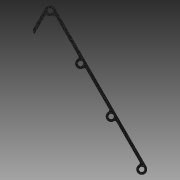
# Autodesk Inventor part: g16-strut2
Saved by Autodesk Inventor 2013 (Build 170138000, 138)
## iProperties
Created: 2013-03-23
Part Number: g16-strut2
Material: Acrylic
Document SubType Name: Modeling
Designer: Beth Scott
Density: 1 g/cm^3
Author: Beth Scott
Autodesk Inventor part; units mm, degrees
ref_plane "YZ Plane" through (0, 0, 0) normal (1, 0, 0) x (0, 1, 0)
ref_plane "XZ Plane" through (0, 0, 0) normal (0, 1, 0) x (-1, 0, 0)
ref_plane "XY Plane" through (0, 0, 0) normal (0, 0, 1) x (1, 0, 0)
sketch "LED Keepout Regions" plane through (0, 0, 0) normal (0, 0, 1) x (1, 0, 0)
  line L0 (115.0132, -121.5492) -> (110.0132, -121.5492) construction
  line L1 (110.0132, -121.5492) -> (110.0132, -116.5492) construction
  line L2 (110.0132, -116.5492) -> (115.0132, -116.5492) construction
  line L3 (115.0132, -116.5492) -> (115.0132, -121.5492) construction
  line L4 (112.5132, -124.1742) -> (112.5132, -113.9242) construction
  line L5 (120.8464, -119.0492) -> (104.1799, -119.0492) construction
  line L6 (109.5132, -122.0492) -> (107.0132, -122.0492) construction
  line L7 (107.0132, -122.0492) -> (107.0132, -116.0492) construction
  line L8 (107.0132, -116.0492) -> (109.5132, -116.0492) construction
  line L9 (109.5132, -116.0492) -> (109.5132, -122.0492) construction
  line L10 (120.8464, -124.1742) -> (104.1799, -124.1742) construction
  line L11 (104.1799, -124.1742) -> (104.1799, -113.9242) construction
  line L12 (104.1799, -113.9242) -> (120.8464, -113.9242) construction
  line L13 (120.8464, -113.9242) -> (120.8464, -124.1742) construction
  line L14 (117.0132, -113.9242) -> (117.0132, -124.1742) construction
  line L15 (105.0132, -113.9242) -> (105.0132, -124.1742) construction
  point P0 (111.5921, -119.1808)
  point P1 (115.0132, -119.0492)
  point P2 (112.5132, -121.5492)
  point P3 (109.5132, -119.0492)
  dimension "LED_StripWidth" = 10.25
  dimension "LED_Package" = 5
  dimension "LED_CapW" = 2.5
  dimension "LED_CapH" = 6
  dimension "d32" = 16.6665
  dimension "d52" = 2
  dimension "d53" = 2
  dimension "LED_CapDist" = 8
  measures "LED_StripWidth" distance of L12.end L10.start
  measures "LED_Package" distance of L0.start L0.end
  measures "LED_CapW" distance of L6.start L6.end
  measures "LED_CapH" distance of L6.end L7.end
  measures "d32" distance of L11.end L12.end
  measures "d52" distance between parallel lines of L7 L15
  measures "d53" distance between parallel lines of L14 L3
  measures "LED_CapDist" distance between parallel lines of L3 L7
sketch "LED Keepout x16" plane through (0, 0, 0) normal (0, 0, 1) x (1, 0, 0)
  line L0 (133.3347, -3) -> (0.0027, -3) construction
  line L1 (116.6682, -31.8672) -> (16.6692, -31.8672) construction
  line L2 (83.3352, -89.6017) -> (50.0022, -89.6017) construction
  line L3 (116.6682, -31.8672) -> (116.6682, -3) construction
  line L4 (100.0017, -60.7344) -> (33.3357, -60.7344) construction
  line L5 (100.0017, -60.7344) -> (100.0017, -31.8672) construction
  line L6 (83.3352, -89.6017) -> (83.3352, -60.7344) construction
  line L7 (66.6687, -118.4689) -> (66.6687, -89.6017) construction
  line L8 (50.0022, -89.6017) -> (50.0022, -3) construction
  line L9 (16.6692, -31.8672) -> (16.6692, -3) construction
  line L10 (33.3357, -60.7344) -> (33.3357, -3) construction
  line L11 (66.6687, -89.6017) -> (66.6687, -3) construction
  line L12 (83.3352, -60.7344) -> (83.3352, -3) construction
  line L13 (100.0017, -31.8672) -> (100.0017, -3) construction
  line L14 (102.5017, -19.9336) -> (97.5017, -19.9336) construction
  line L15 (97.5017, -19.9336) -> (97.5017, -14.9336) construction
  line L16 (97.5017, -14.9336) -> (102.5017, -14.9336) construction
  line L17 (102.5017, -14.9336) -> (102.5017, -19.9336) construction
  line L18 (100.0017, -22.5586) -> (100.0017, -12.3086) construction
  line L19 (108.335, -17.4336) -> (91.6685, -17.4336) construction
  line L20 (97.0017, -20.4336) -> (94.5017, -20.4336) construction
  line L21 (94.5017, -20.4336) -> (94.5017, -14.4336) construction
  line L22 (94.5017, -14.4336) -> (97.0017, -14.4336) construction
  line L23 (97.0017, -14.4336) -> (97.0017, -20.4336) construction
  line L24 (108.335, -22.5586) -> (91.6685, -22.5586) construction
  line L25 (91.6685, -22.5586) -> (91.6685, -12.3086) construction
  line L26 (91.6685, -12.3086) -> (108.335, -12.3086) construction
  line L27 (108.335, -12.3086) -> (108.335, -22.5586) construction
  line L28 (104.5017, -12.3086) -> (104.5017, -22.5586) construction
  line L29 (92.5017, -12.3086) -> (92.5017, -22.5586) construction
  line L30 (85.8352, -19.9336) -> (80.8352, -19.9336) construction
  line L31 (80.8352, -19.9336) -> (80.8352, -14.9336) construction
  line L32 (80.8352, -14.9336) -> (85.8352, -14.9336) construction
  line L33 (85.8352, -14.9336) -> (85.8352, -19.9336) construction
  line L34 (83.3352, -22.5586) -> (83.3352, -12.3086) construction
  line L35 (91.6685, -17.4336) -> (75.002, -17.4336) construction
  line L36 (80.3352, -20.4336) -> (77.8352, -20.4336) construction
  line L37 (77.8352, -20.4336) -> (77.8352, -14.4336) construction
  line L38 (77.8352, -14.4336) -> (80.3352, -14.4336) construction
  line L39 (80.3352, -14.4336) -> (80.3352, -20.4336) construction
  line L40 (91.6685, -22.5586) -> (75.002, -22.5586) construction
  line L41 (75.002, -22.5586) -> (75.002, -12.3086) construction
  line L42 (75.002, -12.3086) -> (91.6685, -12.3086) construction
  line L43 (91.6685, -12.3086) -> (91.6685, -22.5586) construction
  line L44 (87.8352, -12.3086) -> (87.8352, -22.5586) construction
  line L45 (75.8352, -12.3086) -> (75.8352, -22.5586) construction
  line L46 (69.1687, -19.9336) -> (64.1687, -19.9336) construction
  line L47 (64.1687, -19.9336) -> (64.1687, -14.9336) construction
  line L48 (64.1687, -14.9336) -> (69.1687, -14.9336) construction
  line L49 (69.1687, -14.9336) -> (69.1687, -19.9336) construction
  line L50 (66.6687, -22.5586) -> (66.6687, -12.3086) construction
  line L51 (75.002, -17.4336) -> (58.3355, -17.4336) construction
  line L52 (63.6687, -20.4336) -> (61.1687, -20.4336) construction
  line L53 (61.1687, -20.4336) -> (61.1687, -14.4336) construction
  line L54 (61.1687, -14.4336) -> (63.6687, -14.4336) construction
  line L55 (63.6687, -14.4336) -> (63.6687, -20.4336) construction
  line L56 (75.002, -22.5586) -> (58.3355, -22.5586) construction
  line L57 (58.3355, -22.5586) -> (58.3355, -12.3086) construction
  line L58 (58.3355, -12.3086) -> (75.002, -12.3086) construction
  line L59 (75.002, -12.3086) -> (75.002, -22.5586) construction
  line L60 (71.1687, -12.3086) -> (71.1687, -22.5586) construction
  line L61 (59.1687, -12.3086) -> (59.1687, -22.5586) construction
  line L62 (35.8357, -19.9336) -> (30.8357, -19.9336) construction
  line L63 (30.8357, -19.9336) -> (30.8357, -14.9336) construction
  line L64 (30.8357, -14.9336) -> (35.8357, -14.9336) construction
  line L65 (35.8357, -14.9336) -> (35.8357, -19.9336) construction
  line L66 (33.3357, -22.5586) -> (33.3357, -12.3086) construction
  line L67 (41.669, -17.4336) -> (25.0025, -17.4336) construction
  line L68 (30.3357, -20.4336) -> (27.8357, -20.4336) construction
  line L69 (27.8357, -20.4336) -> (27.8357, -14.4336) construction
  line L70 (27.8357, -14.4336) -> (30.3357, -14.4336) construction
  line L71 (30.3357, -14.4336) -> (30.3357, -20.4336) construction
  line L72 (41.669, -22.5586) -> (25.0025, -22.5586) construction
  line L73 (25.0025, -22.5586) -> (25.0025, -12.3086) construction
  line L74 (25.0025, -12.3086) -> (41.669, -12.3086) construction
  line L75 (41.669, -12.3086) -> (41.669, -22.5586) construction
  line L76 (37.8357, -12.3086) -> (37.8357, -22.5586) construction
  line L77 (25.8357, -12.3086) -> (25.8357, -22.5586) construction
  line L78 (52.5022, -19.9336) -> (47.5022, -19.9336) construction
  line L79 (47.5022, -19.9336) -> (47.5022, -14.9336) construction
  line L80 (47.5022, -14.9336) -> (52.5022, -14.9336) construction
  line L81 (52.5022, -14.9336) -> (52.5022, -19.9336) construction
  line L82 (50.0022, -22.5586) -> (50.0022, -12.3086) construction
  line L83 (58.3355, -17.4336) -> (41.669, -17.4336) construction
  line L84 (47.0022, -20.4336) -> (44.5022, -20.4336) construction
  line L85 (44.5022, -20.4336) -> (44.5022, -14.4336) construction
  line L86 (44.5022, -14.4336) -> (47.0022, -14.4336) construction
  line L87 (47.0022, -14.4336) -> (47.0022, -20.4336) construction
  line L88 (58.3355, -22.5586) -> (41.669, -22.5586) construction
  line L89 (41.669, -22.5586) -> (41.669, -12.3086) construction
  line L90 (41.669, -12.3086) -> (58.3355, -12.3086) construction
  line L91 (58.3355, -12.3086) -> (58.3355, -22.5586) construction
  line L92 (54.5022, -12.3086) -> (54.5022, -22.5586) construction
  line L93 (42.5022, -12.3086) -> (42.5022, -22.5586) construction
  line L94 (19.1692, -19.9336) -> (14.1692, -19.9336) construction
  line L95 (14.1692, -19.9336) -> (14.1692, -14.9336) construction
  line L96 (14.1692, -14.9336) -> (19.1692, -14.9336) construction
  line L97 (19.1692, -14.9336) -> (19.1692, -19.9336) construction
  line L98 (16.6692, -22.5586) -> (16.6692, -12.3086) construction
  line L99 (25.0025, -17.4336) -> (8.336, -17.4336) construction
  line L100 (13.6692, -20.4336) -> (11.1692, -20.4336) construction
  line L101 (11.1692, -20.4336) -> (11.1692, -14.4336) construction
  line L102 (11.1692, -14.4336) -> (13.6692, -14.4336) construction
  line L103 (13.6692, -14.4336) -> (13.6692, -20.4336) construction
  line L104 (25.0025, -22.5586) -> (8.336, -22.5586) construction
  line L105 (8.336, -22.5586) -> (8.336, -12.3086) construction
  line L106 (8.336, -12.3086) -> (25.0025, -12.3086) construction
  line L107 (25.0025, -12.3086) -> (25.0025, -22.5586) construction
  line L108 (21.1692, -12.3086) -> (21.1692, -22.5586) construction
  line L109 (9.1692, -12.3086) -> (9.1692, -22.5586) construction
  line L110 (69.1687, -77.6681) -> (64.1687, -77.6681) construction
  line L111 (64.1687, -77.6681) -> (64.1687, -72.6681) construction
  line L112 (64.1687, -72.6681) -> (69.1687, -72.6681) construction
  line L113 (69.1687, -72.6681) -> (69.1687, -77.6681) construction
  line L114 (66.6687, -80.2931) -> (66.6687, -70.0431) construction
  line L115 (75.002, -75.1681) -> (58.3355, -75.1681) construction
  line L116 (63.6687, -78.1681) -> (61.1687, -78.1681) construction
  line L117 (61.1687, -78.1681) -> (61.1687, -72.1681) construction
  line L118 (61.1687, -72.1681) -> (63.6687, -72.1681) construction
  line L119 (63.6687, -72.1681) -> (63.6687, -78.1681) construction
  line L120 (75.002, -80.2931) -> (58.3355, -80.2931) construction
  line L121 (58.3355, -80.2931) -> (58.3355, -70.0431) construction
  line L122 (58.3355, -70.0431) -> (75.002, -70.0431) construction
  line L123 (75.002, -70.0431) -> (75.002, -80.2931) construction
  line L124 (71.1687, -70.0431) -> (71.1687, -80.2931) construction
  line L125 (59.1687, -70.0431) -> (59.1687, -80.2931) construction
  line L126 (52.5022, -77.6681) -> (47.5022, -77.6681) construction
  line L127 (47.5022, -77.6681) -> (47.5022, -72.6681) construction
  line L128 (47.5022, -72.6681) -> (52.5022, -72.6681) construction
  line L129 (52.5022, -72.6681) -> (52.5022, -77.6681) construction
  line L130 (50.0022, -80.2931) -> (50.0022, -70.0431) construction
  line L131 (58.3355, -75.1681) -> (41.669, -75.1681) construction
  line L132 (47.0022, -78.1681) -> (44.5022, -78.1681) construction
  line L133 (44.5022, -78.1681) -> (44.5022, -72.1681) construction
  line L134 (44.5022, -72.1681) -> (47.0022, -72.1681) construction
  line L135 (47.0022, -72.1681) -> (47.0022, -78.1681) construction
  line L136 (58.3355, -80.2931) -> (41.669, -80.2931) construction
  line L137 (41.669, -80.2931) -> (41.669, -70.0431) construction
  line L138 (41.669, -70.0431) -> (58.3355, -70.0431) construction
  line L139 (58.3355, -70.0431) -> (58.3355, -80.2931) construction
  line L140 (54.5022, -70.0431) -> (54.5022, -80.2931) construction
  line L141 (42.5022, -70.0431) -> (42.5022, -80.2931) construction
  line L142 (30.8357, -43.8008) -> (35.8357, -43.8008) construction
  line L143 (35.8357, -43.8008) -> (35.8357, -48.8008) construction
  line L144 (35.8357, -48.8008) -> (30.8357, -48.8008) construction
  line L145 (30.8357, -48.8008) -> (30.8357, -43.8008) construction
  line L146 (33.3357, -41.1758) -> (33.3357, -51.4258) construction
  line L147 (25.0025, -46.3008) -> (41.669, -46.3008) construction
  line L148 (36.3357, -43.3008) -> (38.8357, -43.3008) construction
  line L149 (38.8357, -43.3008) -> (38.8357, -49.3008) construction
  line L150 (38.8357, -49.3008) -> (36.3357, -49.3008) construction
  line L151 (36.3357, -49.3008) -> (36.3357, -43.3008) construction
  line L152 (25.0025, -41.1758) -> (41.669, -41.1758) construction
  line L153 (41.669, -41.1758) -> (41.669, -51.4258) construction
  line L154 (41.669, -51.4258) -> (25.0025, -51.4258) construction
  line L155 (25.0025, -51.4258) -> (25.0025, -41.1758) construction
  line L156 (28.8357, -51.4258) -> (28.8357, -41.1758) construction
  line L157 (40.8357, -51.4258) -> (40.8357, -41.1758) construction
  line L158 (85.8352, -77.6681) -> (80.8352, -77.6681) construction
  line L159 (80.8352, -77.6681) -> (80.8352, -72.6681) construction
  line L160 (80.8352, -72.6681) -> (85.8352, -72.6681) construction
  line L161 (85.8352, -72.6681) -> (85.8352, -77.6681) construction
  line L162 (83.3352, -80.2931) -> (83.3352, -70.0431) construction
  line L163 (91.6685, -75.1681) -> (75.002, -75.1681) construction
  line L164 (80.3352, -78.1681) -> (77.8352, -78.1681) construction
  line L165 (77.8352, -78.1681) -> (77.8352, -72.1681) construction
  line L166 (77.8352, -72.1681) -> (80.3352, -72.1681) construction
  line L167 (80.3352, -72.1681) -> (80.3352, -78.1681) construction
  line L168 (91.6685, -80.2931) -> (75.002, -80.2931) construction
  line L169 (75.002, -80.2931) -> (75.002, -70.0431) construction
  line L170 (75.002, -70.0431) -> (91.6685, -70.0431) construction
  line L171 (91.6685, -70.0431) -> (91.6685, -80.2931) construction
  line L172 (87.8352, -70.0431) -> (87.8352, -80.2931) construction
  line L173 (75.8352, -70.0431) -> (75.8352, -80.2931) construction
  line L174 (64.1687, -43.8008) -> (69.1687, -43.8008) construction
  line L175 (69.1687, -43.8008) -> (69.1687, -48.8008) construction
  line L176 (69.1687, -48.8008) -> (64.1687, -48.8008) construction
  line L177 (64.1687, -48.8008) -> (64.1687, -43.8008) construction
  line L178 (66.6687, -41.1758) -> (66.6687, -51.4258) construction
  line L179 (58.3355, -46.3008) -> (75.002, -46.3008) construction
  line L180 (69.6687, -43.3008) -> (72.1687, -43.3008) construction
  line L181 (72.1687, -43.3008) -> (72.1687, -49.3008) construction
  line L182 (72.1687, -49.3008) -> (69.6687, -49.3008) construction
  line L183 (69.6687, -49.3008) -> (69.6687, -43.3008) construction
  line L184 (58.3355, -41.1758) -> (75.002, -41.1758) construction
  line L185 (75.002, -41.1758) -> (75.002, -51.4258) construction
  line L186 (75.002, -51.4258) -> (58.3355, -51.4258) construction
  line L187 (58.3355, -51.4258) -> (58.3355, -41.1758) construction
  line L188 (62.1687, -51.4258) -> (62.1687, -41.1758) construction
  line L189 (74.1687, -51.4258) -> (74.1687, -41.1758) construction
  line L190 (80.8352, -43.8008) -> (85.8352, -43.8008) construction
  line L191 (85.8352, -43.8008) -> (85.8352, -48.8008) construction
  line L192 (85.8352, -48.8008) -> (80.8352, -48.8008) construction
  line L193 (80.8352, -48.8008) -> (80.8352, -43.8008) construction
  line L194 (83.3352, -41.1758) -> (83.3352, -51.4258) construction
  line L195 (75.002, -46.3008) -> (91.6685, -46.3008) construction
  line L196 (86.3352, -43.3008) -> (88.8352, -43.3008) construction
  line L197 (88.8352, -43.3008) -> (88.8352, -49.3008) construction
  line L198 (88.8352, -49.3008) -> (86.3352, -49.3008) construction
  line L199 (86.3352, -49.3008) -> (86.3352, -43.3008) construction
  line L200 (75.002, -41.1758) -> (91.6685, -41.1758) construction
  line L201 (91.6685, -41.1758) -> (91.6685, -51.4258) construction
  line L202 (91.6685, -51.4258) -> (75.002, -51.4258) construction
  line L203 (75.002, -51.4258) -> (75.002, -41.1758) construction
  line L204 (78.8352, -51.4258) -> (78.8352, -41.1758) construction
  line L205 (90.8352, -51.4258) -> (90.8352, -41.1758) construction
  line L206 (47.5022, -43.8008) -> (52.5022, -43.8008) construction
  line L207 (52.5022, -43.8008) -> (52.5022, -48.8008) construction
  line L208 (52.5022, -48.8008) -> (47.5022, -48.8008) construction
  line L209 (47.5022, -48.8008) -> (47.5022, -43.8008) construction
  line L210 (50.0022, -41.1758) -> (50.0022, -51.4258) construction
  line L211 (41.669, -46.3008) -> (58.3355, -46.3008) construction
  line L212 (53.0022, -43.3008) -> (55.5022, -43.3008) construction
  line L213 (55.5022, -43.3008) -> (55.5022, -49.3008) construction
  line L214 (55.5022, -49.3008) -> (53.0022, -49.3008) construction
  line L215 (53.0022, -49.3008) -> (53.0022, -43.3008) construction
  line L216 (41.669, -41.1758) -> (58.3355, -41.1758) construction
  line L217 (58.3355, -41.1758) -> (58.3355, -51.4258) construction
  line L218 (58.3355, -51.4258) -> (41.669, -51.4258) construction
  line L219 (41.669, -51.4258) -> (41.669, -41.1758) construction
  line L220 (45.5022, -51.4258) -> (45.5022, -41.1758) construction
  line L221 (57.5022, -51.4258) -> (57.5022, -41.1758) construction
  line L222 (97.5017, -43.8008) -> (102.5017, -43.8008) construction
  line L223 (102.5017, -43.8008) -> (102.5017, -48.8008) construction
  line L224 (102.5017, -48.8008) -> (97.5017, -48.8008) construction
  line L225 (97.5017, -48.8008) -> (97.5017, -43.8008) construction
  line L226 (100.0017, -41.1758) -> (100.0017, -51.4258) construction
  line L227 (91.6685, -46.3008) -> (108.335, -46.3008) construction
  line L228 (103.0017, -43.3008) -> (105.5017, -43.3008) construction
  line L229 (105.5017, -43.3008) -> (105.5017, -49.3008) construction
  line L230 (105.5017, -49.3008) -> (103.0017, -49.3008) construction
  line L231 (103.0017, -49.3008) -> (103.0017, -43.3008) construction
  line L232 (91.6685, -41.1758) -> (108.335, -41.1758) construction
  line L233 (108.335, -41.1758) -> (108.335, -51.4258) construction
  line L234 (108.335, -51.4258) -> (91.6685, -51.4258) construction
  line L235 (91.6685, -51.4258) -> (91.6685, -41.1758) construction
  line L236 (95.5017, -51.4258) -> (95.5017, -41.1758) construction
  line L237 (107.5017, -51.4258) -> (107.5017, -41.1758) construction
  line L238 (64.1687, -101.5353) -> (69.1687, -101.5353) construction
  line L239 (69.1687, -101.5353) -> (69.1687, -106.5353) construction
  line L240 (69.1687, -106.5353) -> (64.1687, -106.5353) construction
  line L241 (64.1687, -106.5353) -> (64.1687, -101.5353) construction
  line L242 (66.6687, -98.9103) -> (66.6687, -109.1603) construction
  line L243 (58.3355, -104.0353) -> (75.002, -104.0353) construction
  line L244 (69.6687, -101.0353) -> (72.1687, -101.0353) construction
  line L245 (72.1687, -101.0353) -> (72.1687, -107.0353) construction
  line L246 (72.1687, -107.0353) -> (69.6687, -107.0353) construction
  line L247 (69.6687, -107.0353) -> (69.6687, -101.0353) construction
  line L248 (58.3355, -98.9103) -> (75.002, -98.9103) construction
  line L249 (75.002, -98.9103) -> (75.002, -109.1603) construction
  line L250 (75.002, -109.1603) -> (58.3355, -109.1603) construction
  line L251 (58.3355, -109.1603) -> (58.3355, -98.9103) construction
  line L252 (62.1687, -109.1603) -> (62.1687, -98.9103) construction
  line L253 (74.1687, -109.1603) -> (74.1687, -98.9103) construction
  line L254 (119.1682, -19.9336) -> (114.1682, -19.9336) construction
  line L255 (114.1682, -19.9336) -> (114.1682, -14.9336) construction
  line L256 (114.1682, -14.9336) -> (119.1682, -14.9336) construction
  line L257 (119.1682, -14.9336) -> (119.1682, -19.9336) construction
  line L258 (116.6682, -22.5586) -> (116.6682, -12.3086) construction
  line L259 (125.0015, -17.4336) -> (108.335, -17.4336) construction
  line L260 (113.6682, -20.4336) -> (111.1682, -20.4336) construction
  line L261 (111.1682, -20.4336) -> (111.1682, -14.4336) construction
  line L262 (111.1682, -14.4336) -> (113.6682, -14.4336) construction
  line L263 (113.6682, -14.4336) -> (113.6682, -20.4336) construction
  line L264 (125.0015, -22.5586) -> (108.335, -22.5586) construction
  line L265 (108.335, -22.5586) -> (108.335, -12.3086) construction
  line L266 (108.335, -12.3086) -> (125.0015, -12.3086) construction
  line L267 (125.0015, -12.3086) -> (125.0015, -22.5586) construction
  line L268 (121.1682, -12.3086) -> (121.1682, -22.5586) construction
  line L269 (109.1682, -12.3086) -> (109.1682, -22.5586) construction
  point P0 (73.3279, -41.0278)
  point P1 (116.6682, -17.4336)
  point P2 (116.6682, -17.4336)
  point P3 (100.0017, -17.4336)
  point P4 (100.0017, -17.4336)
  point P5 (83.3352, -75.1681)
  point P6 (100.0017, -46.3008)
  point P7 (66.6687, -104.0353)
  point P8 (83.3352, -17.4336)
  point P9 (66.6687, -17.4336)
  point P10 (33.3357, -17.4336)
  point P11 (16.6692, -17.4336)
  point P12 (100.0017, -46.3008)
  point P13 (83.3352, -46.3008)
  point P14 (66.6687, -46.3008)
  point P15 (50.0022, -46.3008)
  point P16 (33.3357, -46.3008)
  point P17 (50.0022, -75.1681)
  point P18 (66.6687, -75.1681)
  point P19 (83.3352, -75.1681)
  point P20 (66.6687, -104.0353)
  dimension "d56" = 16.6665
  dimension "d61" = 16.6665
  dimension "d62" = 28.8672
  measures "d56" distance from line of L9 L0.end
  measures "d61" distance from line of L0.start L3
  measures "d62" distance of L1.end L9.end
derived "g16-strut1.ipt"
sketch "Strut Templates" plane through (0, 0, 0) normal (0, 1, 0) x (-1, 0, 0)
  circle A0 centre (16.6665, 28.8672) radius 1.5
  circle A1 centre (33.333, 57.7344) radius 1.5
  circle A2 centre (0, 0) radius 1.5
  circle A3 centre (33.333, 0) radius 1.5
  circle A4 centre (66.666, 0) radius 1.5
  circle A5 centre (99.999, 0) radius 1.5
  circle A6 centre (133.332, 0) radius 1.5
  circle A7 centre (116.6655, 28.8672) radius 1.5
  circle A8 centre (99.999, 57.7344) radius 1.5
  circle A9 centre (83.3325, 86.6017) radius 1.5
  circle A10 centre (49.9995, 86.6017) radius 1.5
  circle A11 centre (66.666, 115.4689) radius 1.5
  arc A12 (-2.5981, 1.5) -> (0, -3) centre (0, 0) ccw
  line L0 (0, -3) -> (133.332, -3)
  arc A13 (36.333, 0) -> (30.333, 0) centre (33.333, 0) ccw
  arc A14 (69.666, 0) -> (66.666, -3) centre (66.666, 0) ccw
  circle A15 centre (49.9995, 86.6017) radius 3 construction
  line L1 (-2.5981, 1.5) -> (57.2344, 105.1329)
  circle A16 centre (16.6665, 28.8672) radius 3 construction
  circle A17 centre (33.333, 57.7344) radius 3 construction
  line L2 (29.333, -1) -> (4, -1)
  arc A18 (29.333, -1) -> (30.333, 0) centre (29.333, 0) ccw
  circle A19 centre (0, 0) radius 3 construction
  arc A20 (3, 0) -> (1.5, 2.5981) centre (0, 0) ccw
  arc A21 (3, 0) -> (4, -1) centre (4, 0) ccw
  arc A22 (1.134, 3.9641) -> (1.5, 2.5981) centre (2, 3.4641) ccw
  line L3 (1.134, 3.9641) -> (13.8005, 25.9031)
  arc A23 (15.1665, 26.2691) -> (13.8005, 25.9031) centre (14.6665, 25.4031) ccw
  arc A24 (15.1665, 26.2691) -> (18.1665, 31.4653) centre (16.6665, 28.8672) ccw
  arc A25 (17.8005, 32.8313) -> (18.1665, 31.4653) centre (18.6665, 32.3313) ccw
  line L4 (17.8005, 32.8313) -> (30.467, 54.7703)
  line L5 (34.467, 61.6986) -> (47.1335, 83.6376)
  arc A26 (31.833, 55.1364) -> (34.833, 60.3325) centre (33.333, 57.7344) ccw
  arc A27 (34.467, 61.6986) -> (34.833, 60.3325) centre (35.333, 61.1986) ccw
  arc A28 (31.833, 55.1364) -> (30.467, 54.7703) centre (31.333, 54.2703) ccw
  arc A29 (51.1335, 90.5658) -> (51.4995, 89.1998) centre (51.9995, 90.0658) ccw
  arc A30 (48.4995, 84.0036) -> (51.4995, 89.1998) centre (49.9995, 86.6017) ccw
  arc A31 (48.4995, 84.0036) -> (47.1335, 83.6376) centre (47.9995, 83.1376) ccw
  arc A32 (69.2641, 116.9689) -> (64.0679, 116.9689) centre (66.666, 115.4689) ccw
  line L6 (64.0679, 116.9689) -> (57.235, 105.1339)
  line L7 (51.1335, 90.5658) -> (57.9664, 102.4008)
  line L8 (57.235, 105.1339) -> (57.967, 102.4018)
  line L9 (57.967, 102.4018) -> (63.8, 112.5048)
  line L10 (57.9664, 102.4008) -> (57.2344, 105.1329)
  arc A33 (65.166, 112.8708) -> (68.166, 112.8708) centre (66.666, 115.4689) ccw
  arc A34 (65.166, 112.8708) -> (63.8, 112.5048) centre (64.666, 112.0048) ccw
  arc A35 (133.332, -3) -> (130.332, 0) centre (133.332, 0) ccw
  line L11 (66.666, -3) -> (133.332, -3)
  line L12 (69.2641, 116.9689) -> (119.2636, 30.3672)
  arc A36 (102.999, 0) -> (96.999, 0) centre (99.999, 0) ccw
  arc A37 (131.832, 2.5981) -> (130.332, 0) centre (133.332, 0) ccw
  arc A38 (115.1655, 31.4653) -> (119.2636, 30.3672) centre (116.6655, 28.8672) ccw
  arc A39 (98.499, 60.3325) -> (101.499, 55.1364) centre (99.999, 57.7344) ccw
  arc A40 (81.8325, 89.1998) -> (84.8325, 84.0036) centre (83.3325, 86.6017) ccw
  line L13 (70.666, -1) -> (95.999, -1)
  line L14 (103.999, -1) -> (129.332, -1)
  line L15 (132.198, 3.9641) -> (119.5315, 25.9031)
  line L16 (115.5315, 32.8313) -> (102.865, 54.7703)
  line L17 (98.865, 61.6986) -> (86.1985, 83.6376)
  line L18 (82.1985, 90.5658) -> (69.532, 112.5048)
  arc A41 (69.666, 0) -> (70.666, -1) centre (70.666, 0) ccw
  arc A42 (95.999, -1) -> (96.999, 0) centre (95.999, 0) ccw
  arc A43 (102.999, 0) -> (103.999, -1) centre (103.999, 0) ccw
  arc A44 (129.332, -1) -> (130.332, 0) centre (129.332, 0) ccw
  arc A45 (69.532, 112.5048) -> (68.166, 112.8708) centre (68.666, 112.0048) ccw
  arc A46 (81.8325, 89.1998) -> (82.1985, 90.5658) centre (81.3325, 90.0658) ccw
  arc A47 (86.1985, 83.6376) -> (84.8325, 84.0036) centre (85.3325, 83.1376) ccw
  arc A48 (98.499, 60.3325) -> (98.865, 61.6986) centre (97.999, 61.1986) ccw
  arc A49 (102.865, 54.7703) -> (101.499, 55.1364) centre (101.999, 54.2703) ccw
  arc A50 (119.5315, 25.9031) -> (118.1655, 26.2691) centre (118.6655, 25.4031) ccw
  arc A51 (115.1655, 31.4653) -> (115.5315, 32.8313) centre (114.6655, 32.3313) ccw
  arc A52 (131.832, 2.5981) -> (132.198, 3.9641) centre (131.332, 3.4641) ccw
  line L19 (37.333, -1) -> (62.666, -1)
  arc A53 (36.333, 0) -> (37.333, -1) centre (37.333, 0) ccw
  arc A54 (62.666, -1) -> (63.666, 0) centre (62.666, 0) ccw
  arc A55 (69.666, 0) -> (63.666, 0) centre (66.666, 0) ccw
  line L20 (0, 0) -> (133.332, 0) construction
  line L21 (16.6665, 28.8672) -> (116.6655, 28.8672) construction
  line L22 (49.9995, 86.6017) -> (83.3325, 86.6017) construction
  line L23 (16.6665, 28.8672) -> (16.6665, 0) construction
  line L24 (33.333, 57.7344) -> (99.999, 57.7344) construction
  line L25 (33.333, 57.7344) -> (33.333, 28.8672) construction
  line L26 (49.9995, 86.6017) -> (49.9995, 57.7344) construction
  line L27 (66.666, 115.4689) -> (66.666, 86.6017) construction
  line L28 (83.3325, 86.6017) -> (83.3325, 0) construction
  line L29 (116.6655, 28.8672) -> (116.6655, 0) construction
  line L30 (99.999, 57.7344) -> (99.999, 0) construction
  line L31 (66.666, 86.6017) -> (66.666, 0) construction
  line L32 (49.9995, 57.7344) -> (49.9995, 0) construction
  line L33 (33.333, 28.8672) -> (33.333, 0) construction
  line L34 (30.833, 16.9336) -> (35.833, 16.9336) construction
  line L35 (35.833, 16.9336) -> (35.833, 11.9336) construction
  line L36 (35.833, 11.9336) -> (30.833, 11.9336) construction
  line L37 (30.833, 11.9336) -> (30.833, 16.9336) construction
  line L38 (33.333, 19.5586) -> (33.333, 9.3086) construction
  line L39 (24.9998, 14.4336) -> (41.6663, 14.4336) construction
  line L40 (36.333, 17.4336) -> (38.833, 17.4336) construction
  line L41 (38.833, 17.4336) -> (38.833, 11.4336) construction
  line L42 (38.833, 11.4336) -> (36.333, 11.4336) construction
  line L43 (36.333, 11.4336) -> (36.333, 17.4336) construction
  line L44 (24.9998, 19.5586) -> (41.6663, 19.5586) construction
  line L45 (41.6663, 19.5586) -> (41.6663, 9.3086) construction
  line L46 (41.6663, 9.3086) -> (24.9998, 9.3086) construction
  line L47 (24.9998, 9.3086) -> (24.9998, 19.5586) construction
  line L48 (28.833, 9.3086) -> (28.833, 19.5586) construction
  line L49 (40.833, 9.3086) -> (40.833, 19.5586) construction
  line L50 (47.4995, 16.9336) -> (52.4995, 16.9336) construction
  line L51 (52.4995, 16.9336) -> (52.4995, 11.9336) construction
  line L52 (52.4995, 11.9336) -> (47.4995, 11.9336) construction
  line L53 (47.4995, 11.9336) -> (47.4995, 16.9336) construction
  line L54 (49.9995, 19.5586) -> (49.9995, 9.3086) construction
  line L55 (41.6663, 14.4336) -> (58.3328, 14.4336) construction
  line L56 (52.9995, 17.4336) -> (55.4995, 17.4336) construction
  line L57 (55.4995, 17.4336) -> (55.4995, 11.4336) construction
  line L58 (55.4995, 11.4336) -> (52.9995, 11.4336) construction
  line L59 (52.9995, 11.4336) -> (52.9995, 17.4336) construction
  line L60 (41.6663, 19.5586) -> (58.3328, 19.5586) construction
  line L61 (58.3328, 19.5586) -> (58.3328, 9.3086) construction
  line L62 (58.3328, 9.3086) -> (41.6663, 9.3086) construction
  line L63 (41.6663, 9.3086) -> (41.6663, 19.5586) construction
  line L64 (45.4995, 9.3086) -> (45.4995, 19.5586) construction
  line L65 (57.4995, 9.3086) -> (57.4995, 19.5586) construction
  line L66 (64.166, 16.9336) -> (69.166, 16.9336) construction
  line L67 (69.166, 16.9336) -> (69.166, 11.9336) construction
  line L68 (69.166, 11.9336) -> (64.166, 11.9336) construction
  line L69 (64.166, 11.9336) -> (64.166, 16.9336) construction
  line L70 (66.666, 19.5586) -> (66.666, 9.3086) construction
  line L71 (58.3328, 14.4336) -> (74.9993, 14.4336) construction
  line L72 (69.666, 17.4336) -> (72.166, 17.4336) construction
  line L73 (72.166, 17.4336) -> (72.166, 11.4336) construction
  line L74 (72.166, 11.4336) -> (69.666, 11.4336) construction
  line L75 (69.666, 11.4336) -> (69.666, 17.4336) construction
  line L76 (58.3328, 19.5586) -> (74.9993, 19.5586) construction
  line L77 (74.9993, 19.5586) -> (74.9993, 9.3086) construction
  line L78 (74.9993, 9.3086) -> (58.3328, 9.3086) construction
  line L79 (58.3328, 9.3086) -> (58.3328, 19.5586) construction
  line L80 (62.166, 9.3086) -> (62.166, 19.5586) construction
  line L81 (74.166, 9.3086) -> (74.166, 19.5586) construction
  line L82 (97.499, 16.9336) -> (102.499, 16.9336) construction
  line L83 (102.499, 16.9336) -> (102.499, 11.9336) construction
  line L84 (102.499, 11.9336) -> (97.499, 11.9336) construction
  line L85 (97.499, 11.9336) -> (97.499, 16.9336) construction
  line L86 (99.999, 19.5586) -> (99.999, 9.3086) construction
  line L87 (91.6658, 14.4336) -> (108.3323, 14.4336) construction
  line L88 (102.999, 17.4336) -> (105.499, 17.4336) construction
  line L89 (105.499, 17.4336) -> (105.499, 11.4336) construction
  line L90 (105.499, 11.4336) -> (102.999, 11.4336) construction
  line L91 (102.999, 11.4336) -> (102.999, 17.4336) construction
  line L92 (91.6658, 19.5586) -> (108.3323, 19.5586) construction
  line L93 (108.3323, 19.5586) -> (108.3323, 9.3086) construction
  line L94 (108.3323, 9.3086) -> (91.6658, 9.3086) construction
  line L95 (91.6658, 9.3086) -> (91.6658, 19.5586) construction
  line L96 (95.499, 9.3086) -> (95.499, 19.5586) construction
  line L97 (107.499, 9.3086) -> (107.499, 19.5586) construction
  line L98 (80.8325, 16.9336) -> (85.8325, 16.9336) construction
  line L99 (85.8325, 16.9336) -> (85.8325, 11.9336) construction
  line L100 (85.8325, 11.9336) -> (80.8325, 11.9336) construction
  line L101 (80.8325, 11.9336) -> (80.8325, 16.9336) construction
  line L102 (83.3325, 19.5586) -> (83.3325, 9.3086) construction
  line L103 (74.9993, 14.4336) -> (91.6658, 14.4336) construction
  line L104 (86.3325, 17.4336) -> (88.8325, 17.4336) construction
  line L105 (88.8325, 17.4336) -> (88.8325, 11.4336) construction
  line L106 (88.8325, 11.4336) -> (86.3325, 11.4336) construction
  line L107 (86.3325, 11.4336) -> (86.3325, 17.4336) construction
  line L108 (74.9993, 19.5586) -> (91.6658, 19.5586) construction
  line L109 (91.6658, 19.5586) -> (91.6658, 9.3086) construction
  line L110 (91.6658, 9.3086) -> (74.9993, 9.3086) construction
  line L111 (74.9993, 9.3086) -> (74.9993, 19.5586) construction
  line L112 (78.8325, 9.3086) -> (78.8325, 19.5586) construction
  line L113 (90.8325, 9.3086) -> (90.8325, 19.5586) construction
  line L114 (114.1655, 16.9336) -> (119.1655, 16.9336) construction
  line L115 (119.1655, 16.9336) -> (119.1655, 11.9336) construction
  line L116 (119.1655, 11.9336) -> (114.1655, 11.9336) construction
  line L117 (114.1655, 11.9336) -> (114.1655, 16.9336) construction
  line L118 (116.6655, 19.5586) -> (116.6655, 9.3086) construction
  line L119 (108.3323, 14.4336) -> (124.9988, 14.4336) construction
  line L120 (119.6655, 17.4336) -> (122.1655, 17.4336) construction
  line L121 (122.1655, 17.4336) -> (122.1655, 11.4336) construction
  line L122 (122.1655, 11.4336) -> (119.6655, 11.4336) construction
  line L123 (119.6655, 11.4336) -> (119.6655, 17.4336) construction
  line L124 (108.3323, 19.5586) -> (124.9988, 19.5586) construction
  line L125 (124.9988, 19.5586) -> (124.9988, 9.3086) construction
  line L126 (124.9988, 9.3086) -> (108.3323, 9.3086) construction
  line L127 (108.3323, 9.3086) -> (108.3323, 19.5586) construction
  line L128 (112.1655, 9.3086) -> (112.1655, 19.5586) construction
  line L129 (124.1655, 9.3086) -> (124.1655, 19.5586) construction
  line L130 (64.166, 74.6681) -> (69.166, 74.6681) construction
  line L131 (69.166, 74.6681) -> (69.166, 69.6681) construction
  line L132 (69.166, 69.6681) -> (64.166, 69.6681) construction
  line L133 (64.166, 69.6681) -> (64.166, 74.6681) construction
  line L134 (66.666, 77.2931) -> (66.666, 67.0431) construction
  line L135 (58.3328, 72.1681) -> (74.9993, 72.1681) construction
  line L136 (69.666, 75.1681) -> (72.166, 75.1681) construction
  line L137 (72.166, 75.1681) -> (72.166, 69.1681) construction
  line L138 (72.166, 69.1681) -> (69.666, 69.1681) construction
  line L139 (69.666, 69.1681) -> (69.666, 75.1681) construction
  line L140 (58.3328, 77.2931) -> (74.9993, 77.2931) construction
  line L141 (74.9993, 77.2931) -> (74.9993, 67.0431) construction
  line L142 (74.9993, 67.0431) -> (58.3328, 67.0431) construction
  line L143 (58.3328, 67.0431) -> (58.3328, 77.2931) construction
  line L144 (62.166, 67.0431) -> (62.166, 77.2931) construction
  line L145 (74.166, 67.0431) -> (74.166, 77.2931) construction
  line L146 (80.8325, 74.6681) -> (85.8325, 74.6681) construction
  line L147 (85.8325, 74.6681) -> (85.8325, 69.6681) construction
  line L148 (85.8325, 69.6681) -> (80.8325, 69.6681) construction
  line L149 (80.8325, 69.6681) -> (80.8325, 74.6681) construction
  line L150 (83.3325, 77.2931) -> (83.3325, 67.0431) construction
  line L151 (74.9993, 72.1681) -> (91.6658, 72.1681) construction
  line L152 (86.3325, 75.1681) -> (88.8325, 75.1681) construction
  line L153 (88.8325, 75.1681) -> (88.8325, 69.1681) construction
  line L154 (88.8325, 69.1681) -> (86.3325, 69.1681) construction
  line L155 (86.3325, 69.1681) -> (86.3325, 75.1681) construction
  line L156 (74.9993, 77.2931) -> (91.6658, 77.2931) construction
  line L157 (91.6658, 77.2931) -> (91.6658, 67.0431) construction
  line L158 (91.6658, 67.0431) -> (74.9993, 67.0431) construction
  line L159 (74.9993, 67.0431) -> (74.9993, 77.2931) construction
  line L160 (78.8325, 67.0431) -> (78.8325, 77.2931) construction
  line L161 (90.8325, 67.0431) -> (90.8325, 77.2931) construction
  line L162 (102.499, 40.8008) -> (97.499, 40.8008) construction
  line L163 (97.499, 40.8008) -> (97.499, 45.8008) construction
  line L164 (97.499, 45.8008) -> (102.499, 45.8008) construction
  line L165 (102.499, 45.8008) -> (102.499, 40.8008) construction
  line L166 (99.999, 38.1758) -> (99.999, 48.4258) construction
  line L167 (108.3323, 43.3008) -> (91.6658, 43.3008) construction
  line L168 (96.999, 40.3008) -> (94.499, 40.3008) construction
  line L169 (94.499, 40.3008) -> (94.499, 46.3008) construction
  line L170 (94.499, 46.3008) -> (96.999, 46.3008) construction
  line L171 (96.999, 46.3008) -> (96.999, 40.3008) construction
  line L172 (108.3323, 38.1758) -> (91.6658, 38.1758) construction
  line L173 (91.6658, 38.1758) -> (91.6658, 48.4258) construction
  line L174 (91.6658, 48.4258) -> (108.3323, 48.4258) construction
  line L175 (108.3323, 48.4258) -> (108.3323, 38.1758) construction
  line L176 (104.499, 48.4258) -> (104.499, 38.1758) construction
  line L177 (92.499, 48.4258) -> (92.499, 38.1758) construction
  line L178 (47.4995, 74.6681) -> (52.4995, 74.6681) construction
  line L179 (52.4995, 74.6681) -> (52.4995, 69.6681) construction
  line L180 (52.4995, 69.6681) -> (47.4995, 69.6681) construction
  line L181 (47.4995, 69.6681) -> (47.4995, 74.6681) construction
  line L182 (49.9995, 77.2931) -> (49.9995, 67.0431) construction
  line L183 (41.6663, 72.1681) -> (58.3328, 72.1681) construction
  line L184 (52.9995, 75.1681) -> (55.4995, 75.1681) construction
  line L185 (55.4995, 75.1681) -> (55.4995, 69.1681) construction
  line L186 (55.4995, 69.1681) -> (52.9995, 69.1681) construction
  line L187 (52.9995, 69.1681) -> (52.9995, 75.1681) construction
  line L188 (41.6663, 77.2931) -> (58.3328, 77.2931) construction
  line L189 (58.3328, 77.2931) -> (58.3328, 67.0431) construction
  line L190 (58.3328, 67.0431) -> (41.6663, 67.0431) construction
  line L191 (41.6663, 67.0431) -> (41.6663, 77.2931) construction
  line L192 (45.4995, 67.0431) -> (45.4995, 77.2931) construction
  line L193 (57.4995, 67.0431) -> (57.4995, 77.2931) construction
  line L194 (69.166, 40.8008) -> (64.166, 40.8008) construction
  line L195 (64.166, 40.8008) -> (64.166, 45.8008) construction
  line L196 (64.166, 45.8008) -> (69.166, 45.8008) construction
  line L197 (69.166, 45.8008) -> (69.166, 40.8008) construction
  line L198 (66.666, 38.1758) -> (66.666, 48.4258) construction
  line L199 (74.9993, 43.3008) -> (58.3328, 43.3008) construction
  line L200 (63.666, 40.3008) -> (61.166, 40.3008) construction
  line L201 (61.166, 40.3008) -> (61.166, 46.3008) construction
  line L202 (61.166, 46.3008) -> (63.666, 46.3008) construction
  line L203 (63.666, 46.3008) -> (63.666, 40.3008) construction
  line L204 (74.9993, 38.1758) -> (58.3328, 38.1758) construction
  line L205 (58.3328, 38.1758) -> (58.3328, 48.4258) construction
  line L206 (58.3328, 48.4258) -> (74.9993, 48.4258) construction
  line L207 (74.9993, 48.4258) -> (74.9993, 38.1758) construction
  line L208 (71.166, 48.4258) -> (71.166, 38.1758) construction
  line L209 (59.166, 48.4258) -> (59.166, 38.1758) construction
  line L210 (52.4995, 40.8008) -> (47.4995, 40.8008) construction
  line L211 (47.4995, 40.8008) -> (47.4995, 45.8008) construction
  line L212 (47.4995, 45.8008) -> (52.4995, 45.8008) construction
  line L213 (52.4995, 45.8008) -> (52.4995, 40.8008) construction
  line L214 (49.9995, 38.1758) -> (49.9995, 48.4258) construction
  line L215 (58.3328, 43.3008) -> (41.6663, 43.3008) construction
  line L216 (46.9995, 40.3008) -> (44.4995, 40.3008) construction
  line L217 (44.4995, 40.3008) -> (44.4995, 46.3008) construction
  line L218 (44.4995, 46.3008) -> (46.9995, 46.3008) construction
  line L219 (46.9995, 46.3008) -> (46.9995, 40.3008) construction
  line L220 (58.3328, 38.1758) -> (41.6663, 38.1758) construction
  line L221 (41.6663, 38.1758) -> (41.6663, 48.4258) construction
  line L222 (41.6663, 48.4258) -> (58.3328, 48.4258) construction
  line L223 (58.3328, 48.4258) -> (58.3328, 38.1758) construction
  line L224 (54.4995, 48.4258) -> (54.4995, 38.1758) construction
  line L225 (42.4995, 48.4258) -> (42.4995, 38.1758) construction
  line L226 (85.8325, 40.8008) -> (80.8325, 40.8008) construction
  line L227 (80.8325, 40.8008) -> (80.8325, 45.8008) construction
  line L228 (80.8325, 45.8008) -> (85.8325, 45.8008) construction
  line L229 (85.8325, 45.8008) -> (85.8325, 40.8008) construction
  line L230 (83.3325, 38.1758) -> (83.3325, 48.4258) construction
  line L231 (91.6658, 43.3008) -> (74.9993, 43.3008) construction
  line L232 (80.3325, 40.3008) -> (77.8325, 40.3008) construction
  line L233 (77.8325, 40.3008) -> (77.8325, 46.3008) construction
  line L234 (77.8325, 46.3008) -> (80.3325, 46.3008) construction
  line L235 (80.3325, 46.3008) -> (80.3325, 40.3008) construction
  line L236 (91.6658, 38.1758) -> (74.9993, 38.1758) construction
  line L237 (74.9993, 38.1758) -> (74.9993, 48.4258) construction
  line L238 (74.9993, 48.4258) -> (91.6658, 48.4258) construction
  line L239 (91.6658, 48.4258) -> (91.6658, 38.1758) construction
  line L240 (87.8325, 48.4258) -> (87.8325, 38.1758) construction
  line L241 (75.8325, 48.4258) -> (75.8325, 38.1758) construction
  line L242 (35.833, 40.8008) -> (30.833, 40.8008) construction
  line L243 (30.833, 40.8008) -> (30.833, 45.8008) construction
  line L244 (30.833, 45.8008) -> (35.833, 45.8008) construction
  line L245 (35.833, 45.8008) -> (35.833, 40.8008) construction
  line L246 (33.333, 38.1758) -> (33.333, 48.4258) construction
  line L247 (41.6663, 43.3008) -> (24.9998, 43.3008) construction
  line L248 (30.333, 40.3008) -> (27.833, 40.3008) construction
  line L249 (27.833, 40.3008) -> (27.833, 46.3008) construction
  line L250 (27.833, 46.3008) -> (30.333, 46.3008) construction
  line L251 (30.333, 46.3008) -> (30.333, 40.3008) construction
  line L252 (41.6663, 38.1758) -> (24.9998, 38.1758) construction
  line L253 (24.9998, 38.1758) -> (24.9998, 48.4258) construction
  line L254 (24.9998, 48.4258) -> (41.6663, 48.4258) construction
  line L255 (41.6663, 48.4258) -> (41.6663, 38.1758) construction
  line L256 (37.833, 48.4258) -> (37.833, 38.1758) construction
  line L257 (25.833, 48.4258) -> (25.833, 38.1758) construction
  line L258 (69.166, 98.5353) -> (64.166, 98.5353) construction
  line L259 (64.166, 98.5353) -> (64.166, 103.5353) construction
  line L260 (64.166, 103.5353) -> (69.166, 103.5353) construction
  line L261 (69.166, 103.5353) -> (69.166, 98.5353) construction
  line L262 (66.666, 95.9103) -> (66.666, 106.1603) construction
  line L263 (74.9993, 101.0353) -> (58.3328, 101.0353) construction
  line L264 (63.666, 98.0353) -> (61.166, 98.0353) construction
  line L265 (61.166, 98.0353) -> (61.166, 104.0353) construction
  line L266 (61.166, 104.0353) -> (63.666, 104.0353) construction
  line L267 (63.666, 104.0353) -> (63.666, 98.0353) construction
  line L268 (74.9993, 95.9103) -> (58.3328, 95.9103) construction
  line L269 (58.3328, 95.9103) -> (58.3328, 106.1603) construction
  line L270 (58.3328, 106.1603) -> (74.9993, 106.1603) construction
  line L271 (74.9993, 106.1603) -> (74.9993, 95.9103) construction
  line L272 (71.166, 106.1603) -> (71.166, 95.9103) construction
  line L273 (59.166, 106.1603) -> (59.166, 95.9103) construction
  line L274 (14.1665, 16.9336) -> (19.1665, 16.9336) construction
  line L275 (19.1665, 16.9336) -> (19.1665, 11.9336) construction
  line L276 (19.1665, 11.9336) -> (14.1665, 11.9336) construction
  line L277 (14.1665, 11.9336) -> (14.1665, 16.9336) construction
  line L278 (16.6665, 19.5586) -> (16.6665, 9.3086) construction
  line L279 (8.3333, 14.4336) -> (24.9998, 14.4336) construction
  line L280 (19.6665, 17.4336) -> (22.1665, 17.4336) construction
  line L281 (22.1665, 17.4336) -> (22.1665, 11.4336) construction
  line L282 (22.1665, 11.4336) -> (19.6665, 11.4336) construction
  line L283 (19.6665, 11.4336) -> (19.6665, 17.4336) construction
  line L284 (8.3333, 19.5586) -> (24.9998, 19.5586) construction
  line L285 (24.9998, 19.5586) -> (24.9998, 9.3086) construction
  line L286 (24.9998, 9.3086) -> (8.3333, 9.3086) construction
  line L287 (8.3333, 9.3086) -> (8.3333, 19.5586) construction
  line L288 (12.1665, 9.3086) -> (12.1665, 19.5586) construction
  line L289 (24.1665, 9.3086) -> (24.1665, 19.5586) construction
extrude "Extrusion1" add sketch "Strut Templates" along normal blind 6 contours L6 A32 L12 A38 A51 L16 A49 A39 A48 L17 A47 A40 A46 L18 A45 A33 A34 L9 L8
equation "\"d3\" = ThickLayerThickness"
equation "\"ThickLayerThickness\" = 6"
body "Solid1"
